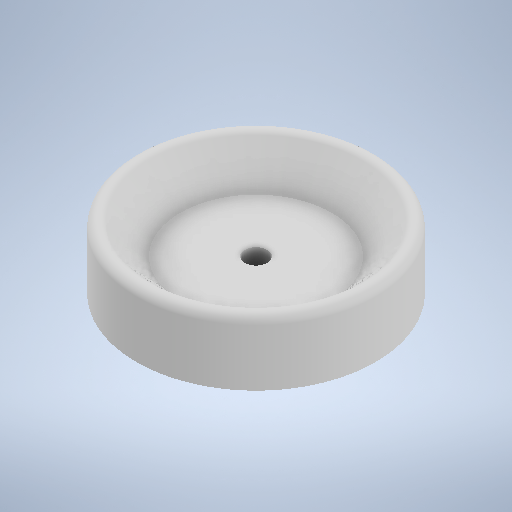
# Autodesk Inventor part: Part1
Saved by Autodesk Inventor 2025 (Build 290162000, 162)
## iProperties
Created: 2024-07-27
Part Number: Part1
Material: Generic
Document SubType Name: Modeling
Designer: ethan
Density: 1 g/cm^3
Appearance: Default
Author: ethan
Autodesk Inventor part; units mm, degrees
ref_plane "YZ Plane" through (0, 0, 0) normal (1, 0, 0) x (0, 1, 0)
ref_plane "XZ Plane" through (0, 0, 0) normal (0, 1, 0) x (-1, 0, 0)
ref_plane "XY Plane" through (0, 0, 0) normal (0, 0, 1) x (1, 0, 0)
sketch "Sketch1" plane through (0, 0, 0) normal (0, 1, 0) x (-1, 0, 0)
  circle A0 centre (0, 0) radius 33.3375
  dimension "d0" = 66.675
  constraints: 1 centre point, 1 coincident
  measures "d0" diameter of A0
extrude "Extrusion1" add sketch "Sketch1" along normal blind 12.7
sketch "Sketch2" plane through (0, 12.7, 0) normal (0, 1, 0) x (1, 0, 0)
  line L0 (0, 0) -> (-3.175, 0)
  line L1 (-3.175, 0) -> (-3.175, 3.175)
  line L2 (-3.175, 3.175) -> (0, 3.175)
  line L3 (0, 3.175) -> (0, 0)
  dimension "d3" = 3.175
  dimension "d4" = 3.175
  constraints: 8 end point, 2 parallel, 1 horizontal, 1 perpendicular
  measures "d3" distance of L0.end L1.end
  measures "d4" distance of L1.end L2.end
extrude "Extrusion2" cut sketch "Sketch2" against normal blind 12.7
sketch "Sketch3" plane through (0, 12.7, -3.175) normal (-1, 0, 0) x (0, 0, 1)
  line L0 (36.5125, 0) -> (-30.1625, 0) projected
  line L1 (36.5125, -12.7) -> (-30.1625, -12.7) projected
  line L2 (0, 0) -> (0, -12.7) projected
  line L3 (3.175, 0) -> (3.175, -12.7) projected
  line L4 (3.175, 0) -> (-47.625, 0)
  line L5 (-30.1625, 0) -> (-47.625, 17.4625)
  line L6 (-30.1625, 0) -> (-5.4668, 0) construction
  line L7 (-47.625, 17.4625) -> (-47.625, -12.7)
  line L8 (36.5125, 0) -> (-30.1625, 0) projected
  line L9 (-47.625, -12.7) -> (-30.1625, -12.7)
  line L10 (-30.1625, 0) -> (-30.1625, -12.7)
  line L11 (-30.1625, -12.7) -> (-30.1625, 0) projected
  line L12 (0, 0) -> (0, 32.402)
  dimension "d8" = 50.8
  dimension "d9" = 135
  constraints: 14 end point, 2 perpendicular, 1 collinear, 1 equal length, 1 horizontal, 1 point on line, 1 vertical
  measures "d8" distance of L3.start L4.end
  measures "d9" angle of L6 L5
revolve "Revolution1" add sketch "Sketch3" angle 360 about axis through (0, 12.7, -3.175) along (0, 1, 0) contours L10 L9 L7 L4 | L4 L7 L5
fillet "Fillet1" radius 3.175 1 edges at (0, 30.1625, 44.45)
sketch "Sketch4" plane through (0, 12.7, -3.175) normal (0, 1, 0) x (1, 0, 0)
  line L0 (0, 0) -> (-3.175, 0) projected
  circle A0 centre (0, 0) radius 4.4901
  point P0 (0, -3.175)
  constraints: 1 centre point
extrude "Extrusion3" cut sketch "Sketch4" against normal blind 12.7
body "Solid1"
